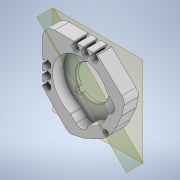
# Autodesk Inventor part: uppermidblock
Saved by Autodesk Inventor 2022 (Build 260153000, 153)
## iProperties
Created: 2022-03-17
Part Number: uppermidblock
Material: Generic
Document SubType Name: Modeling
Designer: zac-h
Density: 1 g/cm^3
Appearance: Default
Author: zac-h
## iProperties of the stored document uppermidblock_3DPrint.ipt
Created: 2022-03-20
Part Number: uppermidblock_3DPrint
Material: Generic
Document SubType Name: Modeling
Designer: zac-h
Density: 1 g/cm^3
Appearance: Default
Author: zac-h
Autodesk Inventor part; units mm, degrees
ref_plane "YZ Plane" through (0, 0, 0) normal (1, 0, 0) x (0, 1, 0)
ref_plane "XZ Plane" through (0, 0, 0) normal (0, 1, 0) x (-1, 0, 0)
ref_plane "XY Plane" through (0, 0, 0) normal (0, 0, 1) x (1, 0, 0)
ref_plane "Work Plane1" through (0, 0, 0) normal (0, 0, 1) x (1, 0, 0)
sketch "Sketch1" plane through (0, 0, 0) normal (0, 0, 1) x (1, 0, 0)
  line L0 (54.6745, 14.0094) -> (51.6007, 0.0667) projected
  arc A0 (54.6745, 14.0094) -> (51.7087, 23.6992) centre (44.6112, 16.228) ccw projected
  line L1 (19.1376, 54.6412) -> (51.7087, 23.6992) projected
  arc A1 (19.1376, 54.6412) -> (18.4488, 54.9162) centre (18.4488, 53.9162) ccw projected
  line L2 (-8.4105, 54.9162) -> (0.0011, 54.9162) projected
  arc A2 (-38.4967, 54.9162) -> (-54.9162, 38.4967) centre (-38.4967, 38.4967) ccw projected
  line L3 (-54.9162, 12.4519) -> (-54.9162, 38.4967) projected
  arc A3 (-54.9162, -18.4488) -> (-54.6412, -19.1376) centre (-53.9162, -18.4488) ccw projected
  line L4 (-23.6992, -51.7087) -> (-54.6412, -19.1376) projected
  arc A4 (-23.6992, -51.7087) -> (-14.0094, -54.6745) centre (-16.228, -44.6112) ccw projected
  line L5 (-0.0667, -51.6007) -> (-14.0094, -54.6745) projected
  arc A5 (-0.0667, -51.6007) -> (0.1266, -51.5369) centre (-0.282, -50.6241) ccw projected
  line L6 (17.6889, -43.6752) -> (0.1266, -51.5369) projected
  line L7 (51.5369, -0.1266) -> (43.6752, -17.6889) projected
  arc A6 (51.5369, -0.1266) -> (51.6007, 0.0667) centre (50.6241, 0.282) ccw projected
  circle A7 centre (-3.3712, 3.3712) radius 22.225
  line L8 (-3.3712, 3.3712) -> (14.5893, 21.3317) construction
  line L9 (-3.3712, 3.3712) -> (22.0288, 3.3712) construction
  circle A8 centre (14.5893, 21.3317) radius 2.132
  circle A9 centre (-21.3317, -14.5893) radius 2.132
  line L10 (-43.8312, 13.1447) -> (-48.5312, 15.8583) projected
  line L11 (-43.8312, 7.7176) -> (-43.8312, 13.1447) projected
  line L12 (-48.5312, 5.0041) -> (-43.8312, 7.7176) projected
  line L13 (-53.2312, 7.7176) -> (-48.5312, 5.0041) projected
  line L14 (-53.2312, 13.1447) -> (-53.2312, 12.4519) projected
  line L15 (-48.5312, 15.8583) -> (-53.2312, 13.1447) projected
  line L16 (-13.1447, 53.2312) -> (-15.8583, 48.5312) projected
  line L17 (-7.7176, 53.2312) -> (-8.4105, 53.2312) projected
  line L18 (-5.0041, 48.5312) -> (-7.7176, 53.2312) projected
  line L19 (-7.7176, 43.8312) -> (-5.0041, 48.5312) projected
  line L20 (-13.1447, 43.8312) -> (-7.7176, 43.8312) projected
  line L21 (-15.8583, 48.5312) -> (-13.1447, 43.8312) projected
  line L22 (-43.8312, 0.4447) -> (-48.5312, 3.1583) projected
  line L23 (-43.8312, -4.9824) -> (-43.8312, 0.4447) projected
  line L24 (-48.5312, -7.6959) -> (-43.8312, -4.9824) projected
  line L25 (-53.2312, -4.9824) -> (-48.5312, -7.6959) projected
  line L26 (-53.2312, 0.4447) -> (-53.2312, -0.2481) projected
  line L27 (-48.5312, 3.1583) -> (-53.2312, 0.4447) projected
  line L28 (-43.8312, -12.2553) -> (-48.5312, -9.5417) projected
  line L29 (-43.8312, -17.6824) -> (-43.8312, -12.2553) projected
  line L30 (-48.5312, -20.3959) -> (-43.8312, -17.6824) projected
  line L31 (-53.2312, -17.6824) -> (-48.5312, -20.3959) projected
  line L32 (-53.2312, -12.2553) -> (-53.2312, -12.9481) projected
  line L33 (-48.5312, -9.5417) -> (-53.2312, -12.2553) projected
  line L34 (-0.4447, 53.2312) -> (-3.1583, 48.5312) projected
  line L35 (4.9824, 53.2312) -> (4.2895, 53.2312) projected
  line L36 (7.6959, 48.5312) -> (4.9824, 53.2312) projected
  line L37 (4.9824, 43.8312) -> (7.6959, 48.5312) projected
  line L38 (-0.4447, 43.8312) -> (4.9824, 43.8312) projected
  line L39 (-3.1583, 48.5312) -> (-0.4447, 43.8312) projected
  line L40 (9.5417, 48.5312) -> (12.2553, 43.8312) projected
  line L41 (12.2553, 53.2312) -> (9.5417, 48.5312) projected
  line L42 (17.6824, 53.2312) -> (16.9895, 53.2312) projected
  line L43 (20.3959, 48.5312) -> (17.6824, 53.2312) projected
  line L44 (17.6824, 43.8312) -> (20.3959, 48.5312) projected
  line L45 (12.2553, 43.8312) -> (17.6824, 43.8312) projected
  circle A10 centre (14.9688, 48.5312) radius 2.132 projected
  circle A11 centre (2.2688, 48.5312) radius 2.132 projected
  circle A12 centre (-10.4312, 48.5312) radius 2.132 projected
  circle A13 centre (-48.5312, 10.4312) radius 2.132 projected
  circle A14 centre (-48.5312, -2.2688) radius 2.132 projected
  circle A15 centre (-48.5312, -14.9688) radius 2.132 projected
  circle A16 centre (30.3259, -30.3259) radius 2.132 projected
  circle A17 centre (-3.3712, 3.3712) radius 39.37 projected
  arc A18 (30.0935, -35.8334) -> (29.6251, -33.7616) centre (29.3145, -34.9207) ccw projected
  line L46 (29.6251, -33.7616) -> (27.4682, -33.1836) projected
  line L47 (27.4682, -33.1836) -> (26.4222, -29.2799) projected
  line L48 (26.4222, -29.2799) -> (29.2799, -26.4222) projected
  line L49 (29.2799, -26.4222) -> (33.1836, -27.4682) projected
  line L50 (33.1836, -27.4682) -> (33.7616, -29.6251) projected
  arc A19 (33.7616, -29.6251) -> (35.8334, -30.0935) centre (34.9207, -29.3145) ccw projected
  arc A20 (35.8334, -30.0935) -> (43.6752, -17.6889) centre (-3.3712, 3.3712) ccw projected
  arc A21 (17.6889, -43.6752) -> (30.0935, -35.8334) centre (-3.3712, 3.3712) ccw projected
  line L51 (11.2743, 24.6467) -> (17.9043, 24.6467)
  line L52 (17.9043, 24.6467) -> (17.9043, 18.0167)
  line L53 (17.9043, 18.0167) -> (11.2743, 18.0167)
  line L54 (11.2743, 18.0167) -> (11.2743, 24.6467)
  line L55 (11.2743, 24.6467) -> (17.9043, 18.0167) construction
  line L56 (17.9043, 24.6467) -> (11.2743, 18.0167) construction
  line L57 (-24.6467, -11.2743) -> (-18.0167, -11.2743)
  line L58 (-18.0167, -11.2743) -> (-18.0167, -17.9043)
  line L59 (-18.0167, -17.9043) -> (-24.6467, -17.9043)
  line L60 (-24.6467, -17.9043) -> (-24.6467, -11.2743)
  line L61 (-24.6467, -11.2743) -> (-18.0167, -17.9043) construction
  line L62 (-18.0167, -11.2743) -> (-24.6467, -17.9043) construction
  line L63 (-12.4519, 53.2312) -> (-12.4519, 54.9162) projected
  line L64 (-38.4967, 54.9162) -> (-12.4519, 54.9162) projected
  line L65 (-54.9162, 12.4519) -> (-53.2312, 12.4519) projected
  line L66 (-53.2312, 8.4105) -> (-53.2312, 7.7176) projected
  line L67 (-53.2312, 8.4105) -> (-54.9162, 8.4105) projected
  line L68 (-54.9162, -0.2481) -> (-54.9162, 8.4105) projected
  line L69 (-54.9162, -0.2481) -> (-53.2312, -0.2481) projected
  line L70 (-53.2312, -4.2895) -> (-53.2312, -4.9824) projected
  line L71 (-53.2312, -4.2895) -> (-54.9162, -4.2895) projected
  line L72 (-54.9162, -12.9481) -> (-54.9162, -4.2895) projected
  line L73 (-54.9162, -12.9481) -> (-53.2312, -12.9481) projected
  line L74 (-53.2312, -16.9895) -> (-53.2312, -17.6824) projected
  line L75 (-53.2312, -16.9895) -> (-54.9162, -16.9895) projected
  line L76 (-54.9162, -18.4488) -> (-54.9162, -16.9895) projected
  line L77 (16.9895, 54.9162) -> (18.4488, 54.9162) projected
  line L78 (16.9895, 54.9162) -> (16.9895, 53.2312) projected
  line L79 (12.9481, 53.2312) -> (12.2553, 53.2312) projected
  line L80 (12.9481, 53.2312) -> (12.9481, 54.9162) projected
  line L81 (4.2895, 54.9162) -> (12.9481, 54.9162) projected
  line L82 (4.2895, 54.9162) -> (4.2895, 53.2312) projected
  line L83 (0.0011, 53.2312) -> (-0.4447, 53.2312) projected
  line L84 (0.0011, 53.2312) -> (0.0011, 54.9162) projected
  line L85 (-8.4105, 54.9162) -> (-8.4105, 53.2312) projected
  line L86 (-12.4519, 53.2312) -> (-13.1447, 53.2312) projected
  point P0 (0, 0)
  point P1 (35.8217, 7.1013)
  point P2 (-4.4886, -35.983)
  point P3 (13.3459, 18.0167)
  point P4 (-18.0167, -13.3459)
  point P5 (-20.0882, -11.2743)
  point P6 (11.2743, 20.0882)
  dimension "d0" = 44.45
  dimension "d1" = 25.4
  dimension "d2" = 45
  dimension "d3" = 4.264
  dimension "d6" = 360
  dimension "d24" = 6.63
  constraints: 28 end point, 4 equal length, 4 midpoint, 4 parallel, 3 centre point, 3 horizontal, 2 coincident, 2 perpendicular, 5 other
  measures "d0" diameter of A7
  measures "d1" distance of L8.start L8.end
  measures "d2" angle of L9 L8
  measures "d3" diameter of A8
  measures "d24" distance of L52.end L53.end
extrude "Extrusion1" add sketch "Sketch1" along normal blind 4 contours L0 A6 L7 A20 A19 L50 L49 L48 L47 L46 A18 A21 L6 A5 L5 A4 L4 A3 L76 L75 L74 L31 L30 L29 L28 L33 L32 L73 L72 L71 L70 L25 L24 L23 L22 L27 L26 L69 L68 L67 L66 L13 L12 L11 L10 L15 L14 L65 L3 A2 L64 L63 L86 L16 L21 L20 L19 L18 L17 L85 L2 L84 L83 L34 L39 L38 L37 L36 L35 L82 L81 L80 L79 L41 L40 L45 L44 L43 L42 L78 L77 A1 L1 A0 | A17
sketch "Sketch2" plane through (0, 0, 4) normal (0, 0, 1) x (1, 0, 0)
  line L0 (0.0011, 54.9162) -> (-8.4105, 54.9162) projected
  arc A0 (-38.4967, 54.9162) -> (-54.9162, 38.4967) centre (-38.4967, 38.4967) ccw projected
  line L1 (-54.9162, 38.4967) -> (-54.9162, 12.4519) projected
  arc A1 (-54.9162, -18.4488) -> (-54.6412, -19.1376) centre (-53.9162, -18.4488) ccw projected
  line L2 (-54.6412, -19.1376) -> (-23.6992, -51.7087) projected
  arc A2 (-23.6992, -51.7087) -> (-14.0094, -54.6745) centre (-16.228, -44.6112) ccw projected
  line L3 (-14.0094, -54.6745) -> (-0.0667, -51.6007) projected
  arc A3 (-0.0667, -51.6007) -> (0.1266, -51.5369) centre (-0.282, -50.6241) ccw projected
  line L4 (0.1266, -51.5369) -> (17.6889, -43.6752) projected
  line L5 (43.6752, -17.6889) -> (51.5369, -0.1266) projected
  arc A4 (51.5369, -0.1266) -> (51.6007, 0.0667) centre (50.6241, 0.282) ccw projected
  line L6 (51.6007, 0.0667) -> (54.6745, 14.0094) projected
  arc A5 (54.6745, 14.0094) -> (51.7087, 23.6992) centre (44.6112, 16.228) ccw projected
  line L7 (51.7087, 23.6992) -> (19.1376, 54.6412) projected
  arc A6 (19.1376, 54.6412) -> (18.4488, 54.9162) centre (18.4488, 53.9162) ccw projected
  circle A7 centre (14.5893, 21.3317) radius 12.7
  circle A8 centre (-21.3317, -14.5893) radius 2.132 projected
  circle A9 centre (14.5893, 21.3317) radius 2.132 projected
  line L8 (14.5893, 21.3317) -> (32.5498, 3.3712) construction
  line L9 (7.8541, 14.5965) -> (25.8146, -3.364)
  line L10 (39.285, 10.1064) -> (21.3245, 28.0669)
  arc A10 (21.3245, 28.0669) -> (7.8541, 14.5965) centre (14.5893, 21.3317) ccw
  arc A11 (25.8146, -3.364) -> (39.285, 10.1064) centre (32.5498, 3.3712) ccw
  line L11 (14.5893, 21.3317) -> (39.9893, 21.3317) construction
  line L12 (-3.3712, 3.3712) -> (-28.0669, 28.0669) construction
  line L13 (-3.3712, 3.3712) -> (31.5538, 3.3712) construction
  circle A12 centre (-21.3317, -14.5893) radius 12.7
  line L14 (-14.5965, -7.8541) -> (3.364, -25.8146)
  line L15 (-10.1064, -39.285) -> (-28.0669, -21.3245)
  arc A13 (-10.1064, -39.285) -> (3.364, -25.8146) centre (-3.3712, -32.5498) ccw
  circle A14 centre (14.9688, 48.5312) radius 2.132 projected
  circle A15 centre (2.2688, 48.5312) radius 2.132 projected
  circle A16 centre (-10.4312, 48.5312) radius 2.132 projected
  line L16 (29.6251, -33.7616) -> (27.4682, -33.1836) projected
  line L17 (27.4682, -33.1836) -> (26.4222, -29.2799) projected
  line L18 (26.4222, -29.2799) -> (29.2799, -26.4222) projected
  line L19 (29.2799, -26.4222) -> (33.1836, -27.4682) projected
  line L20 (33.1836, -27.4682) -> (33.7616, -29.6251) projected
  arc A17 (33.7616, -29.6251) -> (35.8334, -30.0935) centre (34.9207, -29.3145) ccw projected
  arc A18 (35.8334, -30.0935) -> (43.6752, -17.6889) centre (-3.3712, 3.3712) ccw projected
  arc A19 (17.6889, -43.6752) -> (30.0935, -35.8334) centre (-3.3712, 3.3712) ccw projected
  arc A20 (30.0935, -35.8334) -> (29.6251, -33.7616) centre (29.3145, -34.9207) ccw projected
  circle A21 centre (-3.3712, 3.3712) radius 38.1
  circle A22 centre (-48.5312, 10.4312) radius 2.132 projected
  circle A23 centre (-48.5312, -2.2688) radius 2.132 projected
  circle A24 centre (-48.5312, -14.9688) radius 2.132 projected
  line L21 (18.4488, 54.9162) -> (16.9895, 54.9162) projected
  line L22 (16.9895, 54.9162) -> (16.9895, 53.2312) projected
  line L23 (16.9895, 53.2312) -> (17.6824, 53.2312) projected
  line L24 (17.6824, 53.2312) -> (20.3959, 48.5312) projected
  line L25 (20.3959, 48.5312) -> (17.6824, 43.8312) projected
  line L26 (17.6824, 43.8312) -> (12.2553, 43.8312) projected
  line L27 (12.2553, 43.8312) -> (9.5417, 48.5312) projected
  line L28 (9.5417, 48.5312) -> (12.2553, 53.2312) projected
  line L29 (12.2553, 53.2312) -> (12.9481, 53.2312) projected
  line L30 (12.9481, 53.2312) -> (12.9481, 54.9162) projected
  line L31 (12.9481, 54.9162) -> (4.2895, 54.9162) projected
  line L32 (4.2895, 54.9162) -> (4.2895, 53.2312) projected
  line L33 (4.2895, 53.2312) -> (4.9824, 53.2312) projected
  line L34 (4.9824, 53.2312) -> (7.6959, 48.5312) projected
  line L35 (7.6959, 48.5312) -> (4.9824, 43.8312) projected
  line L36 (4.9824, 43.8312) -> (-0.4447, 43.8312) projected
  line L37 (-0.4447, 43.8312) -> (-3.1583, 48.5312) projected
  line L38 (-3.1583, 48.5312) -> (-0.4447, 53.2312) projected
  line L39 (-0.4447, 53.2312) -> (0.0011, 53.2312) projected
  line L40 (0.0011, 53.2312) -> (0.0011, 54.9162) projected
  line L41 (-8.4105, 54.9162) -> (-8.4105, 53.2312) projected
  line L42 (-8.4105, 53.2312) -> (-7.7176, 53.2312) projected
  line L43 (-7.7176, 53.2312) -> (-5.0041, 48.5312) projected
  line L44 (-5.0041, 48.5312) -> (-7.7176, 43.8312) projected
  line L45 (-7.7176, 43.8312) -> (-13.1447, 43.8312) projected
  line L46 (-13.1447, 43.8312) -> (-15.8583, 48.5312) projected
  line L47 (-15.8583, 48.5312) -> (-13.1447, 53.2312) projected
  line L48 (-13.1447, 53.2312) -> (-12.4519, 53.2312) projected
  line L49 (-12.4519, 53.2312) -> (-12.4519, 54.9162) projected
  line L50 (-12.4519, 54.9162) -> (-38.4967, 54.9162) projected
  line L51 (-54.9162, 12.4519) -> (-53.2312, 12.4519) projected
  line L52 (-53.2312, 12.4519) -> (-53.2312, 13.1447) projected
  line L53 (-53.2312, 13.1447) -> (-48.5312, 15.8583) projected
  line L54 (-48.5312, 15.8583) -> (-43.8312, 13.1447) projected
  line L55 (-43.8312, 13.1447) -> (-43.8312, 7.7176) projected
  line L56 (-43.8312, 7.7176) -> (-48.5312, 5.0041) projected
  line L57 (-48.5312, 5.0041) -> (-53.2312, 7.7176) projected
  line L58 (-53.2312, 7.7176) -> (-53.2312, 8.4105) projected
  line L59 (-53.2312, 8.4105) -> (-54.9162, 8.4105) projected
  line L60 (-54.9162, 8.4105) -> (-54.9162, -0.2481) projected
  line L61 (-54.9162, -0.2481) -> (-53.2312, -0.2481) projected
  line L62 (-53.2312, -0.2481) -> (-53.2312, 0.4447) projected
  line L63 (-53.2312, 0.4447) -> (-48.5312, 3.1583) projected
  line L64 (-48.5312, 3.1583) -> (-43.8312, 0.4447) projected
  line L65 (-43.8312, 0.4447) -> (-43.8312, -4.9824) projected
  line L66 (-43.8312, -4.9824) -> (-48.5312, -7.6959) projected
  line L67 (-48.5312, -7.6959) -> (-53.2312, -4.9824) projected
  line L68 (-53.2312, -4.9824) -> (-53.2312, -4.2895) projected
  line L69 (-53.2312, -4.2895) -> (-54.9162, -4.2895) projected
  line L70 (-54.9162, -4.2895) -> (-54.9162, -12.9481) projected
  line L71 (-54.9162, -12.9481) -> (-53.2312, -12.9481) projected
  line L72 (-53.2312, -12.9481) -> (-53.2312, -12.2553) projected
  line L73 (-53.2312, -12.2553) -> (-48.5312, -9.5417) projected
  line L74 (-48.5312, -9.5417) -> (-43.8312, -12.2553) projected
  line L75 (-43.8312, -12.2553) -> (-43.8312, -17.6824) projected
  line L76 (-43.8312, -17.6824) -> (-48.5312, -20.3959) projected
  line L77 (-48.5312, -20.3959) -> (-53.2312, -17.6824) projected
  line L78 (-53.2312, -17.6824) -> (-53.2312, -16.9895) projected
  line L79 (-53.2312, -16.9895) -> (-54.9162, -16.9895) projected
  line L80 (-54.9162, -16.9895) -> (-54.9162, -18.4488) projected
  point P0 (0, 0)
  point P1 (23.5696, 12.3514)
  point P2 (-8.6566, -13.794)
  point P3 (13.794, 8.6566)
  point P4 (27.2644, 22.127)
  point P5 (-22.127, -27.2644)
  point P6 (22.9603, -0.5096)
  point P7 (0.5096, -22.9603)
  point P8 (-30.312, -23.5696)
  point P9 (23.5696, 30.312)
  point P10 (32.0915, 17.2999)
  point P11 (-17.2999, -32.0915)
  point P12 (6.103, -33.5321)
  point P13 (33.5321, -6.103)
  dimension "d10" = 25.4
  dimension "d11" = 25.4
  dimension "d12" = 315
  dimension "d13" = 19.05
  dimension "d14" = 135
  dimension "d23" = 76.2
  constraints: 18 end point, 6 centre point, 6 point on circle, 6 symmetric about line, 4 tangent, 2 equal length, 2 horizontal, 1 coincident, 1 midpoint, 1 parallel, 2 other
  measures "d10" diameter of A7
  measures "d11" distance of L8.start L8.end
  measures "d13" diameter of A11
  measures "d14" angle of L13 L12
  measures "d23" diameter of A21
extrude "Extrusion2" add sketch "Sketch2" along normal blind 15.24 contours L40 L39 L38 L37 L36 L35 L34 L33 L32 L31 L30 L29 L28 L27 L26 L25 L24 L23 L22 L21 A6 L7 A5 L6 A4 L5 A18 A17 L20 L19 L18 L17 L16 A20 A19 L4 A3 L3 A2 L2 A1 L80 L79 L78 L77 L76 L75 L74 L73 L72 L71 L70 L69 L68 L67 L66 L65 L64 L63 L62 L61 L60 L59 L58 L57 L56 L55 L54 L53 L52 L51 L1 A0 L50 L49 L48 L47 L46 L45 L44 L43 L42 L41 L0
ref_plane "Work Plane2" through (-1455.9157, 1455.9157, 0) normal (-0.7071068, -0.7071068, 0) x (0, 0, 1)
fillet "Fillet3" radius 1 4 edges at (13.3459, 18.0167, 2) (11.2743, 20.0882, 2) (-18.0167, -13.3459, 2) (-20.0882, -11.2743, 2)
fillet "Fillet4" radius 3.175 4 edges at (32.0915, 17.2999, 11.62) (33.5321, -6.103, 11.62) (6.103, -33.5321, 11.62) (-17.2999, -32.0915, 11.62)
chamfer "Chamfer3" distance 0.6 angle 45 14 edges at (-21.2739, -10.7285, 4) (-23.4058, -11.2743, 4) (-19.0866, 19.0866, 4) (10.7285, 21.2739, 4) (11.2743, 23.4058, 4) (-24.6467, -14.5893, 4) (-21.3317, -17.9043, 4) (-18.0167, -16.6634, 4) (-17.4708, -14.5315, 4) (12.3443, -12.3443, 4) (14.5315, 17.4708, 4) (16.6634, 18.0167, 4) (17.9043, 21.3317, 4) (14.5893, 24.6467, 4)
sketch "Sketch3" plane through (-1455.9157, 1455.9157, 0) normal (-0.7071068, -0.7071068, 0) x (0, 0, 1)
  line L0 (0, -1988.1137) -> (19.24, -1988.1137) projected
  line L1 (0, -1988.1137) -> (19.24, -2007.3537)
  line L2 (19.24, -2033.1894) -> (19.24, -1992.9228) projected
  line L3 (0, -1988.1137) -> (27.2095, -1988.1137) construction
  line L4 (19.24, -2007.3537) -> (19.24, -1988.1137)
  line L5 (0, -1992.9228) -> (0, -1988.1137) projected
  line L6 (19.24, -1988.1137) -> (0, -1988.1137)
  line L7 (0, -1988.1137) -> (20.631, -1988.1137)
  point P0 (0, -2058.9757)
  point P1 (20.631, -1992.9228)
  point P2 (20.631, -1988.1137)
  dimension "d18" = 45
  constraints: 10 end point, 3 point on line, 1 collinear, 1 equal length, 1 horizontal, 1 perpendicular
  measures "d18" angle of L1 L3
body "Solid1"
